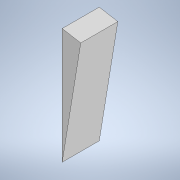
# Autodesk Inventor part: backPlateForLight
Saved by Autodesk Inventor 2021.1 (Build 251245000, 245)
## iProperties
Created: 2020-08-01
Part Number: backPlateForLight
Material: Generic
Document SubType Name: Modeling
Designer: robst
Density: 1 g/cm^3
Appearance: Default
Author: robst
Autodesk Inventor part; units mm, degrees
ref_plane "YZ Plane" through (0, 0, 0) normal (1, 0, 0) x (0, 1, 0)
ref_plane "XZ Plane" through (0, 0, 0) normal (0, 1, 0) x (-1, 0, 0)
ref_plane "XY Plane" through (0, 0, 0) normal (0, 0, 1) x (1, 0, 0)
sketch "Sketch1" plane through (0, 0, 0) normal (0, 0, 1) x (1, 0, 0)
  line L0 (0, 0) -> (0, 79.375)
  line L1 (0, 79.375) -> (12.7, 77.1356)
  line L2 (12.7, 77.1356) -> (0, 0)
  dimension "d0" = 79.375
  dimension "d6" = 80
  dimension "d8" = 12.7
  constraints: 6 end point, 1 vertical
  measures "d0" distance of L0.start L0.end
  measures "d6" angle of L1 L0
  measures "d8" distance from line of L1.end L0
extrude "Extrusion1" add sketch "Sketch1" against normal blind 25.4
sketch "Sketch3" plane through (0, 0, 0) normal (-1, 0, 0) x (0, 0, 1)
  line L0 (-25.4, 77.1356) -> (-25.4, 0) projected
  line L1 (-25.4, 38.5678) -> (0, 38.5678) construction
  line L2 (-14.8227, 41.7428) -> (-17.0097, 35.3928)
  line L3 (-17.0097, 35.3928) -> (-17.9205, 35.3928)
  line L4 (-17.9205, 35.3928) -> (-20.1075, 41.7428)
  line L5 (-20.1075, 41.7428) -> (-19.2018, 41.7428)
  line L6 (-19.2018, 41.7428) -> (-17.4419, 36.4683)
  line L7 (-17.4419, 36.4683) -> (-15.682, 41.7428)
  line L8 (-15.682, 41.7428) -> (-14.8227, 41.7428)
  spline S0 degree 2 poles (-10.3715, 38.5678) (-10.3715, 36.8594) (-11.3646, 35.259) (-12.399, 35.259) knots 0 0 0 1 2 2 2
  spline S1 degree 2 poles (-12.399, 35.259) (-13.4487, 35.259) (-14.4316, 36.8903) (-14.4316, 38.5627) knots 0 0 0 1 2 2 2
  spline S2 degree 2 poles (-14.4316, 38.5627) (-14.4316, 40.2814) (-13.4384, 41.8715) (-12.399, 41.8715) knots 0 0 0 1 2 2 2
  spline S3 degree 2 poles (-12.399, 41.8715) (-11.3544, 41.8715) (-10.3715, 40.2248) (-10.3715, 38.5678) knots 0 0 0 1 2 2 2
  spline S4 degree 2 poles (-11.4624, 36.633) (-11.3389, 36.9469) (-11.236, 37.9143) (-11.236, 38.5678) knots 0 0 0 1 2 2 2
  spline S5 degree 2 poles (-11.236, 38.5678) (-11.236, 39.2213) (-11.3389, 40.1836) (-11.4676, 40.5078) knots 0 0 0 1 2 2 2
  spline S6 degree 2 poles (-11.4676, 40.5078) (-11.5962, 40.832) (-12.0439, 41.1665) (-12.399, 41.1665) knots 0 0 0 1 2 2 2
  spline S7 degree 2 poles (-12.399, 41.1665) (-12.754, 41.1665) (-13.212, 40.832) (-13.3458, 40.4975) knots 0 0 0 1 2 2 2
  spline S8 degree 2 poles (-13.3458, 40.4975) (-13.4745, 40.1733) (-13.5671, 39.1853) (-13.5671, 38.5627) knots 0 0 0 1 2 2 2
  spline S9 degree 2 poles (-13.5671, 38.5627) (-13.5671, 37.8937) (-13.4847, 36.9983) (-13.351, 36.6484) knots 0 0 0 1 2 2 2
  spline S10 degree 2 poles (-13.351, 36.6484) (-13.2275, 36.3191) (-12.7695, 35.964) (-12.399, 35.964) knots 0 0 0 1 2 2 2
  spline S11 degree 2 poles (-12.399, 35.964) (-12.049, 35.964) (-11.5911, 36.2985) (-11.4624, 36.633) knots 0 0 0 1 2 2 2
  line L9 (-5.6424, 35.3928) -> (-9.5584, 35.3928)
  line L10 (-9.5584, 35.3928) -> (-9.5584, 36.2934)
  spline S12 degree 2 poles (-9.5584, 36.2934) (-9.1365, 36.6896) (-8.3852, 37.4254) (-8.025, 37.8217) knots 0 0 0 1 2 2 2
  spline S13 degree 2 poles (-8.025, 37.8217) (-7.2994, 38.6193) (-6.7694, 39.5764) (-6.7694, 40.0859) knots 0 0 0 1 2 2 2
  spline S14 degree 2 poles (-6.7694, 40.0859) (-6.7694, 40.3534) (-6.9341, 40.7548) (-7.0833, 40.8835) knots 0 0 0 1 2 2 2
  spline S15 degree 2 poles (-7.0833, 40.8835) (-7.2325, 41.0121) (-7.6236, 41.1408) (-7.8603, 41.1408) knots 0 0 0 1 2 2 2
  spline S16 degree 2 poles (-7.8603, 41.1408) (-8.0867, 41.1408) (-8.5499, 41.0275) (-8.7608, 40.9401) knots 0 0 0 1 2 2 2
  spline S17 degree 2 poles (-8.7608, 40.9401) (-8.9409, 40.868) (-9.2754, 40.6622) (-9.3783, 40.5901) knots 0 0 0 1 2 2 2
  line L11 (-9.3783, 40.5901) -> (-9.4247, 40.5901)
  line L12 (-9.4247, 40.5901) -> (-9.4247, 41.4958)
  spline S18 degree 2 poles (-9.4247, 41.4958) (-9.1622, 41.6245) (-8.2205, 41.8766) (-7.7986, 41.8766) knots 0 0 0 1 2 2 2
  spline S19 degree 2 poles (-7.7986, 41.8766) (-6.9083, 41.8766) (-5.9049, 40.9349) (-5.9049, 40.1322) knots 0 0 0 1 2 2 2
  spline S20 degree 2 poles (-5.9049, 40.1322) (-5.9049, 39.7565) (-6.0798, 39.1287) (-6.2342, 38.8611) knots 0 0 0 1 2 2 2
  spline S21 degree 2 poles (-6.2342, 38.8611) (-6.3886, 38.5833) (-6.8363, 38.0378) (-7.0833, 37.7754) knots 0 0 0 1 2 2 2
  spline S22 degree 2 poles (-7.0833, 37.7754) (-7.4847, 37.338) (-8.4675, 36.4014) (-8.7608, 36.1287) knots 0 0 0 1 2 2 2
  line L13 (-8.7608, 36.1287) -> (-5.6424, 36.1287)
  line L14 (-5.6424, 36.1287) -> (-5.6424, 35.3928)
  point P0 (0, 0)
  constraints: 2 end point, 2 horizontal, 1 midpoint
extrude "Extrusion3" cut sketch "Sketch3" against normal blind 2.54
body "Solid1"
